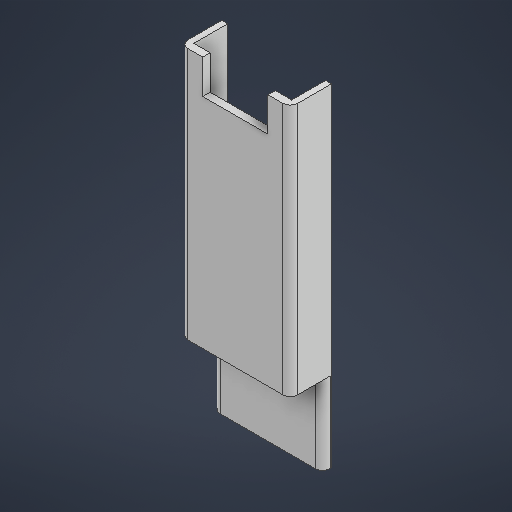
# Autodesk Inventor part: cover^3
Saved by Autodesk Inventor 2025 (Build 290162000, 162)
## iProperties
Created: 2025-02-18
Part Number: cover^3
Material: Generic
Document SubType Name: Modeling
Designer: mayhe
Density: 1 g/cm^3
Appearance: Default
Author: mayhe
Autodesk Inventor part; units mm, degrees
ref_plane "YZ Plane" through (0, 0, 0) normal (1, 0, 0) x (0, 1, 0)
ref_plane "XZ Plane" through (0, 0, 0) normal (0, 1, 0) x (-1, 0, 0)
ref_plane "XY Plane" through (0, 0, 0) normal (0, 0, 1) x (1, 0, 0)
sketch "Sketch1" plane through (0, 0, 0) normal (0, 0, 1) x (1, 0, 0)
  line L0 (-37, 85) -> (37, 85)
  line L1 (37, 85) -> (37, -85)
  line L2 (37, -85) -> (-37, -85)
  line L3 (-37, -85) -> (-37, 85)
  line L4 (-37, 85) -> (37, -85) construction
  line L5 (37, 85) -> (-37, -85) construction
  line L6 (22, 85) -> (-22, 85)
  line L7 (-22, 85) -> (-22, 62)
  line L8 (-22, 62) -> (22, 62)
  line L9 (22, 62) -> (22, 85)
  point P0 (0, 0)
  point P1 (0, 62)
  point P2 (0, 85)
  point P3 (-22, 85)
  dimension "d0" = 74
  dimension "d1" = 170
  dimension "d9" = 44
  dimension "d10" = 23
  constraints: 20 end point, 4 midpoint, 4 parallel, 2 horizontal, 2 perpendicular, 1 point on line, 1 vertical alignment
  measures "d0" distance of L1.end L2.end
  measures "d1" distance of L0.end L1.end
  measures "d9" distance of L8.end L7.end
  measures "d10" distance of L7.end L6.end
extrude "Extrusion1" add sketch "Sketch1" along normal blind 5 contours L0 L7 L8 L9 L1 L2 L3
sketch "Sketch2" plane through (0, 0, 0) normal (0, 0, -1) x (-1, 0, 0)
  circle A0 centre (-26, 81) radius 2.375
  line L0 (0, 0) -> (0, 85)
  line L1 (-37, 85) -> (37, 85) projected
  circle A1 centre (26, 81) radius 2.375
  dimension "d4" = 4.75
  dimension "d5" = 52
  dimension "d8" = 4
  constraints: 2 centre point, 2 end point, 1 midpoint, 1 symmetric about line, 1 other
  measures "d4" diameter of A0
  measures "d5" distance of A1.centre A0.centre
  measures "d8" distance from line of L1 A0.centre
extrude "Extrusion2" cut sketch "Sketch2" against normal blind 4
sketch "Sketch3" plane through (0, 0, 0) normal (0, 0, -1) x (-1, 0, 0)
  line L0 (37, -85) -> (-37, -85) projected
  line L1 (-37, 85) -> (-37, -85)
  line L2 (-37, -85) -> (37, -85)
  line L3 (37, -85) -> (37, 85)
  line L4 (33, 85) -> (33, -81)
  line L5 (33, -81) -> (-33, -81)
  line L6 (-33, -81) -> (-33, 85)
  line L7 (-37, 85) -> (-22, 85) projected
  line L8 (-37, 85) -> (-33, 85)
  line L9 (22, 85) -> (37, 85) projected
  line L10 (33, 85) -> (37, 85)
  line L11 (-33, -81) -> (-27.5, -81)
  line L12 (-27.5, -81) -> (-27.5, -28.7771)
  line L13 (-27.5, -28.7771) -> (-33, -28.7771)
  line L14 (-33, -28.7771) -> (-33, -81)
  line L15 (33, -81) -> (27.5, -81)
  line L16 (27.5, -81) -> (27.5, -28.7771)
  line L17 (27.5, -28.7771) -> (33, -28.7771)
  line L18 (33, -28.7771) -> (33, -81)
  point P0 (0, 0)
  point P1 (33, -28.7771)
  point P2 (-33, -28.7771)
  dimension "d12" = 4
  dimension "d18" = 52.2229
  dimension "d19" = 5.5
  dimension "d20" = 5.5
  constraints: 32 end point, 4 parallel, 3 perpendicular, 2 collinear, 2 horizontal, 1 point on line, 1 vertical, 2 other
  measures "d12" distance between parallel lines of L3 L4
  measures "d18" distance of L12.end L11.end
  measures "d19" distance of L16.end L17.end
  measures "d20" distance between parallel lines of L6 L12
extrude "Extrusion3" add sketch "Sketch3" along normal blind 22.8316
sketch "Sketch4" plane through (-37, -85, 5) normal (0, -1, 0) x (1, 0, 0)
  line L0 (70, -27.8316) -> (74, -27.8316) projected
  line L1 (74, -27.8316) -> (0, -27.8316)
  line L2 (0, -27.8316) -> (0, -21.8316)
  line L3 (0, -21.8316) -> (74, -21.8316)
  line L4 (74, -21.8316) -> (74, -27.8316)
  point P0 (37, -5)
  dimension "d15" = 6
  dimension "d21" = 74
  constraints: 8 end point, 2 parallel, 1 horizontal, 1 perpendicular
  measures "d15" distance of L1.end L2.end
  measures "d21" distance of L0.end L1.end
extrude "Extrusion4" add sketch "Sketch4" along normal blind 54
chamfer "Chamfer1" distance 10 angle 45 2 edges at (30.25, -28.7771, -22.8316) (-30.25, -28.7771, -22.8316)
sketch "Sketch5" plane through (0, 0, -22.8316) normal (0, 0, -1) x (-1, 0, 0)
  line L0 (-31.85, -29.2771) -> (-31.85, -139.7771)
  line L1 (-31.85, -29.2771) -> (78.65, -29.2771) construction
  circle A0 centre (-31.85, -44.2771) radius 2.375
  circle A1 centre (-31.85, -64.2771) radius 2.375
  circle A2 centre (-31.85, -84.2771) radius 2.375
  circle A3 centre (-31.85, -104.2771) radius 2.375
  circle A4 centre (-31.85, -124.2771) radius 2.375
  line L2 (-27.5, -28.7771) -> (-27.5, -81) projected
  line L3 (-37, -85) -> (-37, 85) projected
  line L4 (-27.5, -28.7771) -> (-33, -28.7771) projected
  line L5 (-37, -139) -> (37, -139) projected
  line L6 (0, -139) -> (0, -29.2771)
  circle A5 centre (31.85, -44.2771) radius 2.375
  circle A6 centre (31.85, -64.2771) radius 2.375
  circle A7 centre (31.85, -84.2771) radius 2.375
  circle A8 centre (31.85, -104.2771) radius 2.375
  circle A9 centre (31.85, -124.2771) radius 2.375
  point P0 (0, 0)
  point P1 (-31.85, -36)
  dimension "d23" = 110.5
  dimension "d24" = 90
  dimension "d25" = 4.75
  dimension "d26" = 15
  dimension "d29" = 20
  dimension "d39" = 5.15
  dimension "d40" = 0.5
  constraints: 10 centre point, 6 end point, 5 symmetric about line, 2 perpendicular, 2 point on line, 2 vertical, 1 horizontal, 1 midpoint, 1 vertical alignment, 13 other
  measures "d23" distance of L0.start L0.end
  measures "d24" angle of L0 L1
  measures "d25" diameter of A0
  measures "d26" distance of A0.centre L0.start
  measures "d29" distance of A0.centre A1.centre
  measures "d39" distance between parallel lines of L3 L0
  measures "d40" vertical distance of L2.start L0.start
extrude "Extrusion5" cut sketch "Sketch5" against normal blind 5
fillet "Fillet1" radius 5 4 edges at (37, 0, 5) (-37, 0, 5) (37, -112, -16.8316) (-37, -112, -16.8316)
body "Solid1"
